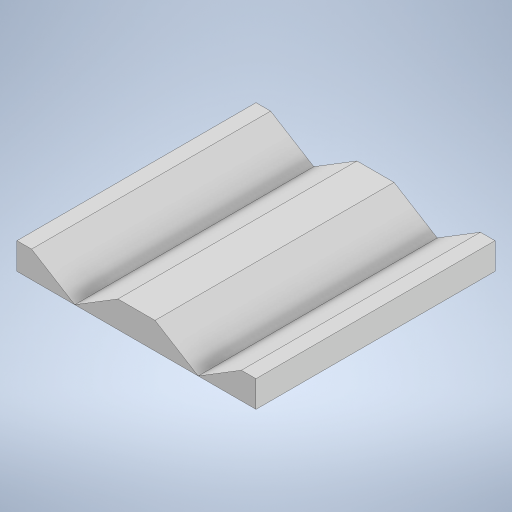
# Autodesk Inventor part: W LandingBase
Saved by Autodesk Inventor 2023 (Build 270158000, 158)
## iProperties
Created: 2022-12-15
Part Number: W LandingBase
Material: Generic
Document SubType Name: Modeling
Designer: ethan
Density: 1 g/cm^3
Appearance: Default
Author: ethan
Autodesk Inventor part; units mm, degrees
ref_plane "YZ Plane" through (0, 0, 0) normal (1, 0, 0) x (0, 1, 0)
ref_plane "XZ Plane" through (0, 0, 0) normal (0, 1, 0) x (-1, 0, 0)
ref_plane "XY Plane" through (0, 0, 0) normal (0, 0, 1) x (1, 0, 0)
sketch "Sketch1" plane through (0, 0, 0) normal (0, 0, 1) x (1, 0, 0)
  line L0 (-247.65, 228.6) -> (-209.55, 228.6)
  line L1 (-209.55, 228.6) -> (-209.55, -228.6)
  line L2 (-209.55, -228.6) -> (-247.65, -228.6)
  line L3 (-247.65, -228.6) -> (-247.65, 228.6)
  line L4 (-228.6, 228.6) -> (-228.6, -228.6) construction
  line L5 (209.55, 228.6) -> (247.65, 228.6)
  line L6 (247.65, 228.6) -> (247.65, -228.6)
  line L7 (247.65, -228.6) -> (209.55, -228.6)
  line L8 (209.55, -228.6) -> (209.55, 228.6)
  line L9 (-349.25, 330.2) -> (349.25, 330.2) construction
  line L10 (349.25, 330.2) -> (349.25, -330.2) construction
  line L11 (349.25, -330.2) -> (-349.25, -330.2) construction
  line L12 (-349.25, -330.2) -> (-349.25, 330.2) construction
  line L13 (-107.95, 228.6) -> (107.95, 228.6) construction
  line L14 (107.95, 228.6) -> (107.95, -228.6) construction
  line L15 (107.95, -228.6) -> (-107.95, -228.6) construction
  line L16 (-107.95, -228.6) -> (-107.95, 228.6) construction
  line L17 (-401.2827, 264.5369) -> (286.6055, 385.8301) construction
  line L18 (286.6055, 385.8301) -> (401.2827, -264.5369) construction
  line L19 (401.2827, -264.5369) -> (-286.6055, -385.8301) construction
  line L20 (-286.6055, -385.8301) -> (-401.2827, 264.5369) construction
  line L21 (-146.006, 206.3817) -> (66.614, 243.8724) construction
  line L22 (66.614, 243.8724) -> (146.006, -206.3817) construction
  line L23 (146.006, -206.3817) -> (-66.614, -243.8724) construction
  line L24 (-66.614, -243.8724) -> (-146.006, 206.3817) construction
  line L25 (-286.6055, 385.8301) -> (401.2827, 264.5369) construction
  line L26 (401.2827, 264.5369) -> (286.6055, -385.8301) construction
  line L27 (286.6055, -385.8301) -> (-401.2827, -264.5369) construction
  line L28 (-401.2827, -264.5369) -> (-286.6055, 385.8301) construction
  line L29 (-66.614, 243.8724) -> (146.006, 206.3817) construction
  line L30 (146.006, 206.3817) -> (66.614, -243.8724) construction
  line L31 (66.614, -243.8724) -> (-146.006, -206.3817) construction
  line L32 (-146.006, -206.3817) -> (-66.614, 243.8724) construction
  line L33 (-401.2827, 385.8301) -> (401.2827, 385.8301)
  line L34 (401.2827, 385.8301) -> (401.2827, -385.8301)
  line L35 (401.2827, -385.8301) -> (-401.2827, -385.8301)
  line L36 (-401.2827, -385.8301) -> (-401.2827, 385.8301)
  line L37 (-457.2, 457.2) -> (457.2, 457.2)
  line L38 (457.2, 457.2) -> (457.2, -457.2)
  line L39 (457.2, -457.2) -> (-457.2, -457.2)
  line L40 (-457.2, -457.2) -> (-457.2, 457.2)
  line L41 (-70.8892, 219.6269) -> (70.8892, 219.6269)
  line L42 (70.8892, 219.6269) -> (70.8892, -219.6269)
  line L43 (70.8892, -219.6269) -> (-70.8892, -219.6269)
  line L44 (-70.8892, -219.6269) -> (-70.8892, 219.6269)
  circle A0 centre (0, 0) radius 480.6325 construction
  circle A1 centre (0, 0) radius 252.8066 construction
  point P0 (228.6, 228.6)
  point P1 (-70.8892, 219.6269)
  point P2 (-70.8892, -219.6269)
  point P3 (0, -385.8301)
  point P4 (0, 385.8301)
  point P5 (70.8892, 219.6269)
  point P6 (70.8892, 219.6269)
  dimension "d0" = 38.1
  dimension "d1" = 457.2
  dimension "d2" = 228.6
  dimension "d4" = 228.6
  dimension "d5" = 38.1
  dimension "d6" = 457.2
  dimension "d7" = 228.6
  dimension "d8" = 228.6
  dimension "d9" = 101.6
  dimension "d10" = 101.6
  dimension "d11" = 101.6
  dimension "d12" = 101.6
  dimension "d23" = 241.3
  dimension "d24" = 241.3
  dimension "d25" = 101.6
  dimension "d26" = 101.6
  dimension "d27" = 241.3
  dimension "d28" = 241.3
  dimension "d29" = 101.6
  dimension "d30" = 101.6
  dimension "d31" = 241.3
  dimension "d32" = 241.3
  dimension "d33" = 101.6
  dimension "d34" = 101.6
  dimension "d35" = 914.4
  dimension "d36" = 914.4
  dimension "d37" = 71.3698
  dimension "d38" = 802.5655
  dimension "d39" = 771.6603
  dimension "d40" = 55.9173
  dimension "d43" = 330.3936
  constraints: 90 end point, 22 parallel, 16 point on line, 11 perpendicular, 7 horizontal, 5 midpoint, 1 coincident, 14 other
  measures "d0" distance of L1.end L2.end
  measures "d1" distance of L0.end L1.end
  measures "d2" distance from line of point (0, 0) L4
  measures "d4" horizontal distance of point (0, 0) L4.start
  measures "d5" distance of L6.end L7.end
  measures "d6" distance of L5.end L6.end
  measures "d7" horizontal distance of point (0, 0) point (228.6, 228.6)
  measures "d8" horizontal distance of point (0, 0) point (228.6, 228.6)
  measures "d9" distance between parallel lines of L3 L12
  measures "d10" distance between parallel lines of L10 L6
  measures "d11" distance between parallel lines of L11 L7
  measures "d12" distance between parallel lines of L9 L5
  measures "d23" distance between parallel lines of L16 L12
  measures "d24" distance between parallel lines of L10 L14
  measures "d25" distance between parallel lines of L11 L15
  measures "d26" distance between parallel lines of L9 L13
  measures "d27" distance between parallel lines of L24 L20
  measures "d28" distance between parallel lines of L18 L22
  measures "d29" distance between parallel lines of L19 L23
  measures "d30" distance between parallel lines of L17 L21
  measures "d31" distance between parallel lines of L32 L28
  measures "d32" distance between parallel lines of L26 L30
  measures "d33" distance between parallel lines of L27 L31
  measures "d34" distance between parallel lines of L25 L29
  measures "d35" distance of L39.end L37.start
  measures "d36" distance of L37.start L37.end
  measures "d37" distance between parallel lines of L35 L39
  measures "d38" distance of L33.start L33.end
  measures "d39" distance of L33.end L34.end
  measures "d40" distance between parallel lines of L40 L36
  measures "d43" distance between parallel lines of L44 L36
extrude "Extrusion1" add sketch "Sketch1" along normal blind 101.6 contours L0 L1 L2 L3 | L5 L6 L7 L8 | L33 L34 L35 L36 | L37 L38 L39 L40 | L41 L42 L43 L44
sketch "Sketch2" plane through (-457.2, -457.2, 0) normal (0, -1, 0) x (1, 0, 0)
  line L0 (0, 101.6) -> (914.4, 101.6) projected
  line L1 (0, 101.6) -> (55.9054, 101.6)
  line L2 (55.9054, 101.6) -> (386.3086, 101.6) construction
  line L3 (914.4, 101.6) -> (858.4946, 101.6)
  line L4 (858.4946, 101.6) -> (528.0914, 101.6) construction
  line L5 (0, 0) -> (914.4, 0) projected
  line L6 (221.107, 101.6) -> (221.107, 0) construction
  line L7 (693.293, 101.6) -> (693.293, 0) construction
  line L8 (55.9054, 101.6) -> (221.107, 0)
  line L9 (858.4946, 101.6) -> (693.293, 0)
  line L10 (528.0914, 101.6) -> (693.293, 0)
  line L11 (386.3086, 101.6) -> (221.107, 0)
  line L12 (386.3086, 101.6) -> (528.0914, 101.6)
  line L13 (55.9054, 101.6) -> (386.3086, 101.6)
  line L14 (528.0914, 101.6) -> (858.4946, 101.6)
  point P0 (457.2, 0)
  dimension "d46" = 55.9054
  dimension "d47" = 330.4032
  dimension "d48" = 55.9054
  dimension "d49" = 330.4032
  constraints: 26 end point, 6 point on line, 3 collinear, 2 midpoint, 2 perpendicular
  measures "d46" distance of L0.start L1.end
  measures "d47" distance of L1.end L2.end
  measures "d48" distance of L0.end L3.end
  measures "d49" distance of L3.end L4.end
extrude "Extrusion2" cut sketch "Sketch2" against normal up to next contours L0 L11 L8 | L0 L9 L10
equation "\"d5\" = d0"
equation "\"d6\" = d1"
equation "\"d7\" = d4"
equation "\"d8\" = d2"
body "Solid1"
